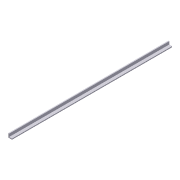
# Autodesk Inventor part: FE-00006-09
Saved by Autodesk Inventor 2012 (Build 160160000, 160)
## iProperties
Created: 2008-05-25
Part Number: FE-00006-09
Document SubType Name: Modeling
Designer: firstuser
Density: 1 g/cm^3
Mass: 301.112 g
Surface Area: 1089.51 cm^2
Volume: 301.112 cm^3
Material: Default
Author: firstuser
Autodesk Inventor part; units mm, degrees
ref_plane "YZ Plane" through (0, 0, 0) normal (1, 0, 0) x (0, 1, 0)
ref_plane "XZ Plane" through (0, 0, 0) normal (0, 1, 0) x (-1, 0, 0)
ref_plane "XY Plane" through (0, 0, 0) normal (0, 0, 1) x (1, 0, 0)
sketch "Sketch1" plane through (0, 0, 0) normal (0, 0, 1) x (1, 0, 0)
  line L0 (-13.5788, 21.5446) -> (-13.5788, -3.8554)
  line L1 (-13.5788, -3.8554) -> (11.8212, -3.8554)
  line L2 (11.8212, -3.8554) -> (11.8212, 2.4946)
  line L3 (11.8212, 2.4946) -> (-7.2288, 2.4946)
  line L4 (-7.2288, 2.4946) -> (-7.2288, 21.5446)
  line L5 (-7.2288, 21.5446) -> (-13.5788, 21.5446)
  dimension "d0" = 25.4
  dimension "d1" = 25.4
  dimension "d2" = 6.35
  constraints: 12 end point, 3 parallel, 2 perpendicular, 1 vertical
  measures "d0" distance of L0.start L0.end
  measures "d1" distance of L0.end L1.end
  measures "d2" distance between parallel lines of L0 L4
extrude "Extrusion1" add sketch "Sketch1" along normal blind 1066.8
body "Solid1"
